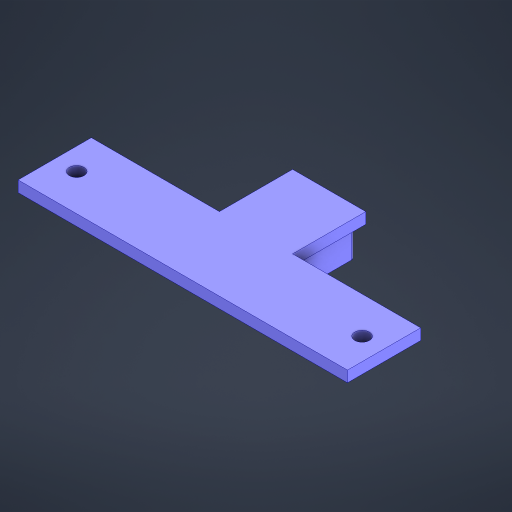
# Autodesk Inventor part: bumper
Saved by Autodesk Inventor 2024 (Build 280153000, 153)
## iProperties
Created: 2023-05-10
Part Number: bumper
Material: Типовые
Document SubType Name: Modeling
Designer: user
Density: 1 g/cm^3
Appearance: По умолчанию
Author: user
Autodesk Inventor part; units mm, degrees
ref_plane "YZ Plane" through (0, 0, 0) normal (1, 0, 0) x (0, 1, 0)
ref_plane "XZ Plane" through (0, 0, 0) normal (0, 1, 0) x (-1, 0, 0)
ref_plane "XY Plane" through (0, 0, 0) normal (0, 0, 1) x (1, 0, 0)
sketch "Эскиз1" plane through (0, 0, 0) normal (0, 0, 1) x (1, 0, 0)
  line L0 (0, 0) -> (90, 0)
  line L1 (90, 0) -> (90, 20)
  line L2 (0, 20) -> (0, 0)
  circle A0 centre (6, 10) radius 2
  circle A1 centre (84, 10) radius 2
  line L3 (0, 20) -> (35, 20)
  line L4 (35, 20) -> (35, 40)
  line L5 (35, 40) -> (55, 40)
  line L6 (55, 40) -> (55, 20)
  line L7 (55, 20) -> (90, 20)
  point P0 (0, 10)
  point P1 (90, 10)
  point P2 (45, 40)
  point P3 (45, 0)
  dimension "d0" = 6
  dimension "d1" = 6
  dimension "d2" = 4
  dimension "d3" = 4
  dimension "d4" = 20
  dimension "d40" = 90
  dimension "d41" = 20
  constraints: 16 end point, 6 perpendicular, 4 midpoint, 2 centre point, 2 horizontal, 2 horizontal alignment, 1 parallel, 1 point on line, 1 vertical alignment
  measures "d0" horizontal distance of L2.start A0.centre
  measures "d1" horizontal distance of L1.end A1.centre
  measures "d2" diameter of A1
  measures "d3" diameter of A0
  measures "d4" distance of L0.start L2.start
  measures "d40" distance of L0.end L0.start
  measures "d41" distance of L4.end L5.end
extrude "Выдавливание1" add sketch "Эскиз1" along normal blind 3
sketch "Эскиз5" plane through (0, 0, 0) normal (0, 0, -1) x (-1, 0, 0)
  line L0 (-53.5, 38.5) -> (-36.5, 38.5)
  line L1 (-36.5, 38.5) -> (-36.5, 21.5)
  line L2 (-36.5, 21.5) -> (-53.5, 21.5)
  line L3 (-53.5, 21.5) -> (-53.5, 38.5)
  line L4 (-35, 40) -> (-35, 20) projected
  line L5 (-55, 40) -> (-35, 40) projected
  point P0 (0, 0)
  point P1 (-45, 38.5)
  point P2 (-45, 40)
  dimension "d46" = 1.5
  dimension "d47" = 1.5
  dimension "d48" = 1.5
  constraints: 8 end point, 2 midpoint, 2 parallel, 1 horizontal, 1 perpendicular, 1 vertical alignment
  measures "d46" distance from line of L4 L0.end
  measures "d47" horizontal distance of L4.start L0.end
  measures "d48" horizontal distance of L1.end L4.end
extrude "Выдавливание4" add sketch "Эскиз5" along normal blind 8
shell "Оболочка2" thickness 2 removed faces 1 at (42.1667, 32.8333, -8)
fillet "Сопряжение3" radius 1 4 edges at (36.5, 38.5, -4) (36.5, 21.5, -4) (53.5, 38.5, -4) (53.5, 21.5, -4)
equation "\"d1\" = d0"
equation "\"d3\" = d2"
